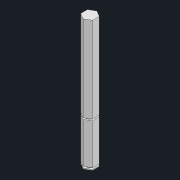
# Autodesk Inventor part: Wasp Pivot Axle
Saved by Autodesk Inventor 2022 (Build 260153000, 153)
## iProperties
Created: 2022-09-18
Part Number: Wasp Pivot Axle
Material: Generic
Document SubType Name: Modeling
Designer: robpl
Density: 1 g/cm^3
Appearance: Default
Author: robpl
Autodesk Inventor part; units mm, degrees
ref_plane "YZ Plane" through (0, 0, 0) normal (1, 0, 0) x (0, 1, 0)
ref_plane "XZ Plane" through (0, 0, 0) normal (0, 1, 0) x (-1, 0, 0)
ref_plane "XY Plane" through (0, 0, 0) normal (0, 0, 1) x (1, 0, 0)
sketch "Sketch1" plane through (0, 0, 0) normal (0, 1, 0) x (-1, 0, 0)
  line L0 (6.35, 3.6662) -> (6.35, -3.6662)
  line L1 (6.35, -3.6662) -> (0, -7.3323)
  line L2 (0, -7.3323) -> (-6.35, -3.6662)
  line L3 (-6.35, -3.6662) -> (-6.35, 3.6662)
  line L4 (-6.35, 3.6662) -> (0, 7.3323)
  line L5 (0, 7.3323) -> (6.35, 3.6662)
  point P0 (0, 0)
  point P1 (0, 0)
  dimension "d0" = 12.7
  constraints: 12 end point, 1 coincident, 1 vertical, 13 other
  measures "d0" distance between parallel lines of L3 L0
extrude "Extrusion1" add sketch "Sketch1" along normal blind 140
sketch "Sketch2" plane through (0, 0, 0) normal (0, 0, 1) x (1, 0, 0)
  line L0 (-15, 1) -> (-5, 1)
  line L1 (-5, 1) -> (-5, 2.5)
  line L2 (-5, 2.5) -> (-15, 2.5)
  line L3 (-15, 2.5) -> (-15, 1)
  line L4 (0, 0) -> (0, 140) projected
  line L5 (0, 0) -> (6.35, 0) projected
  line L6 (0, -26) -> (0, 156) projected
  line L7 (-15, 46) -> (-5, 46)
  line L8 (-5, 46) -> (-5, 47.5)
  line L9 (-5, 47.5) -> (-15, 47.5)
  line L10 (-15, 47.5) -> (-15, 46)
  point P0 (-15, 46.75)
  dimension "d3" = 1.5
  dimension "d4" = 10
  dimension "d5" = 5
  dimension "d6" = 1
  dimension "d8" = 43.5
  constraints: 16 end point, 4 parallel, 2 equal length, 2 horizontal, 2 perpendicular, 1 coincident, 1 midpoint, 1 vertical alignment
  measures "d3" distance of L2.end L0.start
  measures "d4" distance of L0.start L0.end
  measures "d5" distance between parallel lines of L4 L1
  measures "d6" distance from line of L0 L4.start
  measures "d8" distance between parallel lines of L2 L7
revolve "Revolution1" cut sketch "Sketch2" angle 360 about axis through (0, -10, 0) along (0, 1, 0)
body "Solid1"
